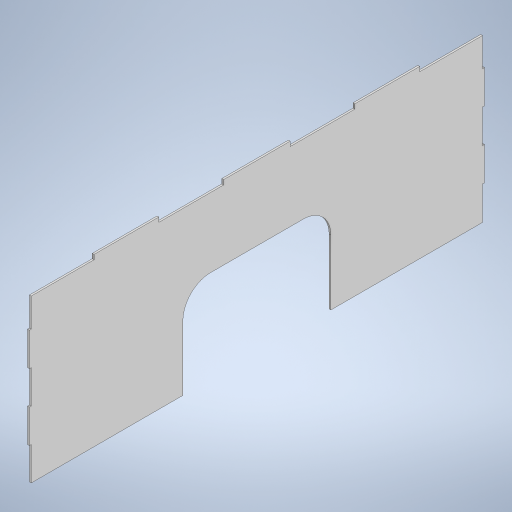
# Autodesk Inventor part: outer_side
Saved by Autodesk Inventor 2023 (Build 270158000, 158)
## iProperties
Created: 2023-04-26
Part Number: outer_side
Material: Generic
Document SubType Name: Modeling
Designer: Unnar
Density: 1 g/cm^3
Appearance: Default
Author: Unnar
Autodesk Inventor part; units mm, degrees
ref_plane "YZ Plane" through (0, 0, 0) normal (1, 0, 0) x (0, 1, 0)
ref_plane "XZ Plane" through (0, 0, 0) normal (0, 1, 0) x (-1, 0, 0)
ref_plane "XY Plane" through (0, 0, 0) normal (0, 0, 1) x (1, 0, 0)
sketch "Sketch1" plane through (0, 0, 0) normal (1, 0, 0) x (0, 1, 0)
  line L0 (98.4407, 261.352) -> (-81.5593, 261.352)
  line L1 (-81.5593, -230.648) -> (98.4407, -230.648)
  line L2 (98.4407, -230.648) -> (98.4407, 261.352)
  line L3 (-81.5593, 95.352) -> (-11.5593, 95.352)
  line L4 (18.4407, 65.352) -> (18.4407, -34.648)
  line L5 (-11.5593, -64.648) -> (-81.5593, -64.648)
  line L6 (-81.5593, 261.352) -> (-81.5593, 95.352)
  line L7 (-81.5593, -64.648) -> (-81.5593, -230.648)
  arc A0 (18.4407, 65.352) -> (-11.5593, 95.352) centre (-11.5593, 65.352) ccw
  arc A1 (-11.5593, -64.648) -> (18.4407, -34.648) centre (-11.5593, -34.648) ccw
  point P0 (0, 0)
  point P1 (18.4407, -64.648)
  point P2 (18.4407, 95.352)
  dimension "d0" = 180
  dimension "d1" = 492
  dimension "d2" = 100
  dimension "d3" = 160
  dimension "d4" = 166
  dimension "d5" = 100
  dimension "d8" = 30
  constraints: 16 end point, 4 parallel, 4 point on circle, 4 point on line, 4 tangent, 3 perpendicular, 2 centre point, 2 horizontal, 1 equal radius
  measures "d0" distance of L0.start L0.end
  measures "d1" distance of L1.end L0.start
  measures "d2" distance of L3.start point (18.441, 95.352)
  measures "d3" distance of point (18.441, 95.352) point (18.441, -64.648)
  measures "d4" distance between parallel lines of L0 L3
  measures "d5" distance of point (18.441, -64.648) L5.end
  measures "d8" radius of A0
extrude "Extrusion1" add sketch "Sketch1" along normal blind 2
sketch "Sketch2" plane through (2, 0, 0) normal (1, 0, 0) x (0, 0, -1)
  line L0 (-261.352, 98.4407) -> (-191.352, 98.4407)
  line L1 (-191.352, 98.4407) -> (-191.352, 93.4407)
  line L2 (-191.352, 93.4407) -> (-261.352, 93.4407)
  line L3 (-261.352, 93.4407) -> (-261.352, 98.4407)
  line L4 (230.648, 98.4407) -> (-261.352, 98.4407) projected
  line L5 (-121.352, 98.4407) -> (-51.352, 98.4407)
  line L6 (-51.352, 98.4407) -> (-51.352, 93.4407)
  line L7 (-51.352, 93.4407) -> (-121.352, 93.4407)
  line L8 (-121.352, 93.4407) -> (-121.352, 98.4407)
  line L9 (20.648, 98.4407) -> (90.648, 98.4407)
  line L10 (90.648, 98.4407) -> (90.648, 93.4407)
  line L11 (90.648, 93.4407) -> (20.648, 93.4407)
  line L12 (20.648, 93.4407) -> (20.648, 98.4407)
  line L13 (160.648, 98.4407) -> (230.648, 98.4407)
  line L14 (230.648, 98.4407) -> (230.648, 93.4407)
  line L15 (230.648, 93.4407) -> (160.648, 93.4407)
  line L16 (160.648, 93.4407) -> (160.648, 98.4407)
  line L17 (230.648, -81.5593) -> (230.648, 98.4407) projected
  point P0 (0, 0)
  point P1 (230.648, 95.9407)
  point P2 (90.648, 95.9407)
  dimension "d9" = 70
  dimension "d10" = 70
  dimension "d11" = 70
  dimension "d12" = 70
  dimension "d13" = 0
  dimension "d14" = 70
  dimension "d15" = 70
  dimension "d16" = 72
  dimension "d17" = 5
  constraints: 32 end point, 8 parallel, 6 point on line, 4 horizontal, 4 perpendicular, 2 midpoint
  measures "d9" distance of L1.end L2.end
  measures "d10" distance between parallel lines of L8 L1
  measures "d11" distance of L6.end L7.end
  measures "d12" distance of L14.end L15.end
  measures "d13" distance from line of L17 point (230.648, 95.941)
  measures "d14" distance from line of point (90.648, 95.941) L16
  measures "d15" distance of L10.end L11.end
  measures "d16" distance between parallel lines of L12 L6
  measures "d17" distance between parallel lines of L2 L0
extrude "Extrusion2" cut sketch "Sketch2" against normal blind 2
sketch "Sketch3" plane through (2, 0, 0) normal (1, 0, 0) x (0, 0, -1)
  line L0 (-261.352, 93.4407) -> (-261.352, -81.5593) projected
  line L1 (-261.352, 93.4407) -> (-259.352, 93.4407)
  line L2 (-259.352, 93.4407) -> (-259.352, 62.4407)
  line L3 (-259.352, 62.4407) -> (-261.352, 62.4407)
  line L4 (-261.352, 62.4407) -> (-261.352, 93.4407)
  line L5 (-261.352, 26.4407) -> (-259.352, 26.4407)
  line L6 (-259.352, 26.4407) -> (-259.352, -9.5593)
  line L7 (-259.352, -9.5593) -> (-261.352, -9.5593)
  line L8 (-261.352, -9.5593) -> (-261.352, 26.4407)
  line L9 (-261.352, -81.5593) -> (-259.352, -81.5593)
  line L10 (-259.352, -81.5593) -> (-259.352, -45.5593)
  line L11 (-259.352, -45.5593) -> (-261.352, -45.5593)
  line L12 (-261.352, -45.5593) -> (-261.352, -81.5593)
  line L13 (64.648, -81.5593) -> (230.648, -81.5593) projected
  line L14 (230.648, -81.5593) -> (228.648, -81.5593)
  line L15 (228.648, -81.5593) -> (228.648, -45.5593)
  line L16 (228.648, -45.5593) -> (230.648, -45.5593)
  line L17 (230.648, -45.5593) -> (230.648, -81.5593)
  line L18 (230.648, -81.5593) -> (230.648, 93.4407) projected
  line L19 (230.648, -9.5593) -> (228.648, -9.5593)
  line L20 (228.648, -9.5593) -> (228.648, 26.4407)
  line L21 (228.648, 26.4407) -> (230.648, 26.4407)
  line L22 (230.648, 26.4407) -> (230.648, -9.5593)
  line L23 (160.648, 93.4407) -> (230.648, 93.4407) projected
  line L24 (230.648, 62.4407) -> (228.648, 62.4407)
  line L25 (228.648, 62.4407) -> (228.648, 93.4407)
  line L26 (228.648, 93.4407) -> (230.648, 93.4407)
  line L27 (230.648, 93.4407) -> (230.648, 62.4407)
  point P0 (0, 0)
  point P1 (-260.352, -9.5593)
  point P2 (-260.352, -45.5593)
  point P3 (-260.352, 62.4407)
  point P4 (-260.352, 26.4407)
  point P5 (229.648, 26.4407)
  point P6 (229.648, 62.4407)
  point P7 (229.648, -9.5593)
  point P8 (229.648, -45.5593)
  dimension "d20" = 36
  dimension "d21" = 36
  dimension "d22" = 36
  dimension "d23" = 36
  dimension "d24" = 2
  dimension "d25" = 2
  dimension "d26" = 36
  dimension "d27" = 36
  dimension "d28" = 36
  dimension "d29" = 36
  constraints: 48 end point, 12 parallel, 8 midpoint, 8 point on line, 6 horizontal, 6 perpendicular
  measures "d20" distance of L9.end L10.end
  measures "d21" distance of L5.end L6.end
  measures "d22" distance of point (-260.352, -9.559) point (-260.352, -45.559)
  measures "d23" distance of point (-260.352, 62.441) point (-260.352, 26.441)
  measures "d24" distance between parallel lines of L0 L2
  measures "d25" distance between parallel lines of L18 L15
  measures "d26" distance of L14.end L15.end
  measures "d27" distance of L19.end L20.end
  measures "d28" distance of point (229.648, 26.441) point (229.648, 62.441)
  measures "d29" distance of point (229.648, -9.559) point (229.648, -45.559)
extrude "Extrusion3" cut sketch "Sketch3" against normal blind 2
body "Solid1"
